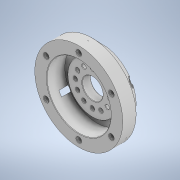
# Autodesk Inventor part: TopFlywheelClamp
Saved by Autodesk Inventor 2020 (Build 240168000, 168)
## iProperties
Created: 2020-02-07
Part Number: TopFlywheelClamp
Material: Generic
Document SubType Name: Modeling
Designer: srini
Density: 1 g/cm^3
Appearance: Default
Author: srini
Autodesk Inventor part; units mm, degrees
ref_plane "YZ Plane" through (0, 0, 0) normal (1, 0, 0) x (0, 1, 0)
ref_plane "XZ Plane" through (0, 0, 0) normal (0, 1, 0) x (-1, 0, 0)
sketch "Sketch1" plane through (0, 0, 0) normal (0, 0, 1) x (1, 0, 0)
  circle A0 centre (0, 0) radius 61.2775
  dimension "d0" = 122.555
  constraints: 1 centre point, 1 coincident
  measures "d0" diameter of A0
extrude "Extrusion1" add sketch "Sketch1" along normal blind 31.242
sketch "Sketch2" plane through (0, 0, 31.242) normal (0, 0, 1) x (1, 0, 0)
  circle A0 centre (0, 0) radius 44.577
  circle A1 centre (0, 0) radius 34.798
  dimension "d3" = 69.596
  dimension "d4" = 89.154
  constraints: 2 centre point, 2 coincident
  measures "d3" diameter of A1
  measures "d4" diameter of A0
extrude "Extrusion2" cut sketch "Sketch2" against normal blind 25.146
sketch "Sketch3" plane through (0, 0, 31.242) normal (0, 0, 1) x (1, 0, 0)
  circle A0 centre (0, 0) radius 34.798 projected
extrude "Extrusion3" cut sketch "Sketch3" against normal blind 19.05
chamfer "Chamfer1" distance 12.7 angle 45 1 edges at (-61.2775, 0, 0)
ref_plane "Work Plane1" through (0, 0, 18.542) normal (0, 0, 1) x (1, 0, 0)
sketch "Sketch5" plane through (0, 0, 18.542) normal (0, 0, 1) x (1, 0, 0)
  circle A0 centre (0, 52.3875) radius 3.3734
  circle A1 centre (-45.3689, 26.1938) radius 3.3734
  circle A2 centre (-45.3689, -26.1938) radius 3.3734
  circle A3 centre (0, -52.3875) radius 3.3734
  circle A4 centre (45.3689, -26.1938) radius 3.3734
  circle A5 centre (45.3689, 26.1937) radius 3.3734
  point P0 (0, 0)
  dimension "d13" = 52.3875
  dimension "d16" = 360
  dimension "d18" = 6.7469
  constraints: 6 centre point, 1 vertical alignment, 13 other
  measures "d13" distance of A0.centre point (0, 0)
  measures "d18" diameter of A0
extrude "Extrusion4" cut sketch "Sketch5" against normal through all both and the other way through all
sketch "Sketch6" plane through (0, 0, 18.542) normal (0, 0, 1) x (1, 0, 0)
  circle A0 centre (-45.3689, 26.1938) radius 3.3734 projected
  line L0 (-48.5768, 20.6375) -> (-51.7847, 26.1938)
  line L1 (-51.7847, 26.1938) -> (-48.5768, 31.75)
  line L2 (-48.5768, 31.75) -> (-42.161, 31.75)
  line L3 (-42.161, 31.75) -> (-38.9531, 26.1938)
  line L4 (-38.9531, 26.1938) -> (-42.161, 20.6375)
  line L5 (-42.161, 20.6375) -> (-48.5768, 20.6375)
  line L6 (-50.1808, 28.9719) -> (-40.5571, 23.4156) construction
  line L7 (6.4158, -52.3875) -> (3.2079, -57.9438)
  line L8 (3.2079, -57.9438) -> (-3.2079, -57.9438)
  line L9 (-3.2079, -57.9438) -> (-6.4158, -52.3875)
  line L10 (-6.4158, -52.3875) -> (-3.2079, -46.8313)
  line L11 (-3.2079, -46.8313) -> (3.2079, -46.8313)
  line L12 (3.2079, -46.8313) -> (6.4158, -52.3875)
  line L13 (0, -57.9438) -> (0, -46.8313) construction
  line L14 (42.161, 31.75) -> (48.5768, 31.75)
  line L15 (48.5768, 31.75) -> (51.7847, 26.1937)
  line L16 (51.7847, 26.1937) -> (48.5768, 20.6375)
  line L17 (48.5768, 20.6375) -> (42.161, 20.6375)
  line L18 (42.161, 20.6375) -> (38.9531, 26.1937)
  line L19 (38.9531, 26.1937) -> (42.161, 31.75)
  line L20 (50.1808, 28.9719) -> (40.5571, 23.4156) construction
  circle A1 centre (-45.3689, -26.1938) radius 3.3734 projected
  circle A2 centre (-45.3689, -26.1938) radius 8.763
  circle A3 centre (45.3689, -26.1938) radius 8.763
  circle A4 centre (0, 52.3875) radius 8.763
  point P0 (0, 0)
  point P1 (-42.4559, 27.8951)
  point P2 (-45.3858, 22.8204)
  point P3 (0, -52.3875)
  point P4 (0, 0)
  point P5 (45.3689, 26.1937)
  point P6 (0, 0)
  dimension "d21" = 11.1125
  dimension "d24" = 360
  dimension "d28" = 17.526
  dimension "d31" = 360
  constraints: 42 end point, 4 coincident, 3 centre point, 3 point on line, 2 midpoint, 71 other
  measures "d21" distance between parallel lines of L1 L4
  measures "d28" diameter of A2
extrude "Extrusion5" cut sketch "Sketch6" against normal through all contours A0 | L0 L1 L2 L3 L4 L5 | L7 L8 L9 L10 L11 L12 | L14 L15 L16 L17 L18 L19 | A1 | A2 | A3 | A4
sketch "Sketch8" plane through (0, 0, 0) normal (0, 0, -1) x (-1, 0, 0)
  circle A0 centre (0, 0) radius 14.3002
  circle A1 centre (0, -23.8125) radius 2.5797
  circle A2 centre (11.9062, -20.6222) radius 2.5797
  circle A3 centre (20.6222, -11.9063) radius 2.5797
  circle A4 centre (23.8125, 0) radius 2.5797
  circle A5 centre (20.6222, 11.9062) radius 2.5797
  circle A6 centre (11.9063, 20.6222) radius 2.5797
  circle A7 centre (0, 23.8125) radius 2.5797
  circle A8 centre (-11.9062, 20.6222) radius 2.5797
  circle A9 centre (-20.6222, 11.9063) radius 2.5797
  circle A10 centre (-23.8125, 0) radius 2.5797
  circle A11 centre (-20.6222, -11.9062) radius 2.5797
  circle A12 centre (-11.9063, -20.6222) radius 2.5797
  dimension "d33" = 28.6004
  dimension "d34" = 5.1594
  dimension "d35" = 23.8125
  dimension "d38" = 360
  constraints: 13 centre point, 1 coincident, 1 vertical alignment, 25 other
  measures "d33" diameter of A0
  measures "d34" diameter of A1
  measures "d35" distance of point (0, 0) A1.centre
extrude "Extrusion6" cut sketch "Sketch8" against normal through all
chamfer "Chamfer2" distance 0.635 angle 45 34 edges at (14.3002, 0, 0) (2.5797, -23.8125, 0) (-9.3266, -20.6222, 0) (-18.0425, -11.9063, 0) (-21.2328, 0, 0) (-18.0425, 11.9062, 0) (-9.3266, 20.6222, 0) (2.5797, 23.8125, 0) (14.4859, 20.6222, 0) (23.2019, 11.9063, 0) (26.3922, 0, 0) (23.2019, -11.9062, 0) (14.4859, -20.6222, 0) (-34.798, 0, 12.192) (-44.577, 0, 31.242) (-48.7423, 26.1938, 31.242) (-3.3734, 52.3875, 31.242) (41.9955, 26.1937, 31.242) (41.9955, -26.1938, 31.242) (-3.3734, -52.3875, 31.242) (-48.7423, -26.1938, 31.242) (2.5797, 23.8125, 12.192) (-9.3266, 20.6222, 12.192) (-18.0425, 11.9062, 12.192) (-21.2328, 0, 12.192) (-18.0425, -11.9063, 12.192) (-9.3266, -20.6222, 12.192) (2.5797, -23.8125, 12.192) (14.4859, -20.6222, 12.192) (23.2019, -11.9062, 12.192) (26.3922, 0, 12.192) (23.2019, 11.9063, 12.192) (14.4859, 20.6222, 12.192) (14.3002, 0, 12.192)
sketch "Sketch9" plane through (0, 0, 18.542) normal (0, 0, -1) x (-1, 0, 0)
  line L0 (46.8289, -16.9181) -> (38.0659, -32.096)
  line L1 (38.0659, -32.096) -> (43.9089, -35.4694)
  line L2 (43.9089, -35.4694) -> (52.6719, -20.2915)
  line L3 (52.6719, -20.2915) -> (46.8289, -16.9181)
  circle A0 centre (45.3689, -26.1938) radius 3.3734 projected
  line L4 (46.8289, -16.9181) -> (43.9089, -35.4694) construction
  line L5 (38.0659, -32.096) -> (52.6719, -20.2915) construction
  line L6 (48.2904, -27.8805) -> (42.4474, -24.507) construction
  circle A1 centre (45.3689, -26.1938) radius 3.3734 projected
  line L7 (38.0659, 32.096) -> (46.8289, 16.9181)
  line L8 (46.8289, 16.9181) -> (52.6719, 20.2915)
  line L9 (52.6719, 20.2915) -> (43.9089, 35.4694)
  line L10 (43.9089, 35.4694) -> (38.0659, 32.096)
  line L11 (38.0659, 32.096) -> (52.6719, 20.2915) construction
  line L12 (46.8289, 16.9181) -> (43.9089, 35.4694) construction
  line L13 (48.2904, 27.8805) -> (42.4474, 24.507) construction
  line L14 (-8.763, 49.0141) -> (8.763, 49.0141)
  line L15 (8.763, 49.0141) -> (8.763, 55.7609)
  line L16 (8.763, 55.7609) -> (-8.763, 55.7609)
  line L17 (-8.763, 55.7609) -> (-8.763, 49.0141)
  line L18 (-8.763, 49.0141) -> (8.763, 55.7609) construction
  line L19 (8.763, 49.0141) -> (-8.763, 55.7609) construction
  line L20 (0, 55.7609) -> (0, 49.0141) construction
  line L21 (-46.8289, 16.9181) -> (-38.0659, 32.096)
  line L22 (-38.0659, 32.096) -> (-43.9089, 35.4694)
  line L23 (-43.9089, 35.4694) -> (-52.6719, 20.2915)
  line L24 (-52.6719, 20.2915) -> (-46.8289, 16.9181)
  line L25 (-46.8289, 16.9181) -> (-43.9089, 35.4694) construction
  line L26 (-38.0659, 32.096) -> (-52.6719, 20.2915) construction
  line L27 (-48.2904, 27.8805) -> (-42.4474, 24.507) construction
  line L28 (-38.0659, -32.096) -> (-46.8289, -16.9181)
  line L29 (-46.8289, -16.9181) -> (-52.6719, -20.2915)
  line L30 (-52.6719, -20.2915) -> (-43.9089, -35.4694)
  line L31 (-43.9089, -35.4694) -> (-38.0659, -32.096)
  line L32 (-38.0659, -32.096) -> (-52.6719, -20.2915) construction
  line L33 (-46.8289, -16.9181) -> (-43.9089, -35.4694) construction
  line L34 (-48.2904, -27.8805) -> (-42.4474, -24.507) construction
  line L35 (8.763, -49.0141) -> (-8.763, -49.0141)
  line L36 (-8.763, -49.0141) -> (-8.763, -55.7609)
  line L37 (-8.763, -55.7609) -> (8.763, -55.7609)
  line L38 (8.763, -55.7609) -> (8.763, -49.0141)
  line L39 (8.763, -49.0141) -> (-8.763, -55.7609) construction
  line L40 (-8.763, -49.0141) -> (8.763, -55.7609) construction
  line L41 (0, -55.7609) -> (0, -49.0141) construction
  point P0 (0, 0)
  point P1 (45.3425, -17.4308)
  point P2 (37.7667, -30.5524)
  point P3 (0, 0)
  point P4 (0, 0)
  point P5 (0, 0)
  point P6 (0, 0)
  point P7 (0, 0)
  point P8 (44.2466, -34.8846)
  point P9 (52.3342, -20.8764)
  dimension "d47" = 360
  constraints: 84 end point, 6 point on line, 4 midpoint, 2 coincident, 2 parallel, 1 perpendicular, 1 tangent, 85 other
extrude "Extrusion7" cut sketch "Sketch9" against normal blind 0.3
sketch "Sketch10" plane through (0, 0, 18.842) normal (0, 0, -1) x (-1, 0, 0)
  line L0 (44.1341, -21.5855) -> (40.7607, -27.4285)
  line L1 (40.7607, -27.4285) -> (46.6037, -30.802)
  line L2 (46.6037, -30.802) -> (49.9771, -24.959)
  line L3 (49.9771, -24.959) -> (44.1341, -21.5855)
  circle A0 centre (45.3689, -26.1938) radius 4.0084 construction
  line L4 (44.1341, -21.5855) -> (46.6037, -30.802) construction
  line L5 (40.7607, -27.4285) -> (49.9771, -24.959) construction
  line L6 (48.2904, -27.8805) -> (42.4474, -24.507) construction
  arc A1 (42.4474, -24.507) -> (48.2904, -27.8805) centre (45.3689, -26.1938) ccw projected
  line L7 (40.7607, 27.4285) -> (44.1341, 21.5855)
  line L8 (44.1341, 21.5855) -> (49.9771, 24.959)
  line L9 (49.9771, 24.959) -> (46.6037, 30.802)
  line L10 (46.6037, 30.802) -> (40.7607, 27.4285)
  line L11 (40.7607, 27.4285) -> (49.9771, 24.959) construction
  line L12 (44.1341, 21.5855) -> (46.6037, 30.802) construction
  line L13 (48.2904, 27.8805) -> (42.4474, 24.507) construction
  line L14 (-3.3734, 49.0141) -> (3.3734, 49.0141)
  line L15 (3.3734, 49.0141) -> (3.3734, 55.7609)
  line L16 (3.3734, 55.7609) -> (-3.3734, 55.7609)
  line L17 (-3.3734, 55.7609) -> (-3.3734, 49.0141)
  line L18 (-3.3734, 49.0141) -> (3.3734, 55.7609) construction
  line L19 (3.3734, 49.0141) -> (-3.3734, 55.7609) construction
  line L20 (0, 55.7609) -> (0, 49.0141) construction
  line L21 (-44.1341, 21.5855) -> (-40.7607, 27.4285)
  line L22 (-40.7607, 27.4285) -> (-46.6037, 30.802)
  line L23 (-46.6037, 30.802) -> (-49.9771, 24.959)
  line L24 (-49.9771, 24.959) -> (-44.1341, 21.5855)
  line L25 (-44.1341, 21.5855) -> (-46.6037, 30.802) construction
  line L26 (-40.7607, 27.4285) -> (-49.9771, 24.959) construction
  line L27 (-48.2904, 27.8805) -> (-42.4474, 24.507) construction
  line L28 (-40.7607, -27.4285) -> (-44.1341, -21.5855)
  line L29 (-44.1341, -21.5855) -> (-49.9771, -24.959)
  line L30 (-49.9771, -24.959) -> (-46.6037, -30.802)
  line L31 (-46.6037, -30.802) -> (-40.7607, -27.4285)
  line L32 (-40.7607, -27.4285) -> (-49.9771, -24.959) construction
  line L33 (-44.1341, -21.5855) -> (-46.6037, -30.802) construction
  line L34 (-48.2904, -27.8805) -> (-42.4474, -24.507) construction
  line L35 (3.3734, -49.0141) -> (-3.3734, -49.0141)
  line L36 (-3.3734, -49.0141) -> (-3.3734, -55.7609)
  line L37 (-3.3734, -55.7609) -> (3.3734, -55.7609)
  line L38 (3.3734, -55.7609) -> (3.3734, -49.0141)
  line L39 (3.3734, -49.0141) -> (-3.3734, -55.7609) construction
  line L40 (-3.3734, -49.0141) -> (3.3734, -55.7609) construction
  line L41 (0, -55.7609) -> (0, -49.0141) construction
  point P0 (0, 0)
  point P1 (0, 0)
  point P2 (42.4474, 24.507)
  point P3 (48.2904, 27.8805)
  point P4 (0, 0)
  point P5 (0, 49.0141)
  point P6 (0, 55.7609)
  point P7 (0, 0)
  point P8 (-42.4474, 24.507)
  point P9 (-48.2904, 27.8805)
  point P10 (0, 0)
  point P11 (-42.4474, -24.507)
  point P12 (-48.2904, -27.8805)
  point P13 (0, 0)
  point P14 (0, -49.0141)
  point P15 (0, -55.7609)
  dimension "d53" = 360
  constraints: 84 end point, 6 point on line, 4 midpoint, 2 coincident, 2 parallel, 2 tangent, 1 perpendicular, 95 other
extrude "Extrusion8" cut sketch "Sketch10" against normal blind 0.3
body "Solid1"
